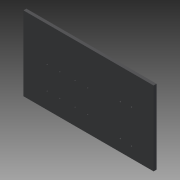
# Autodesk Inventor part: Base
Saved by Autodesk Inventor 2014 SP2 (Build 180246200, 246)
## iProperties
Created: 2015-09-24
Part Number: Base
Material: PVC, non plastifié
Document SubType Name: Modeling
Designer: sd
Density: 1.4 g/cm^3
Appearance: Gris
Mass: 783.12 g
Surface Area: 1491.46 cm^2
Volume: 559.372 cm^3
Author: sd
Autodesk Inventor part; units mm, degrees
ref_plane "YZ Plane" through (0, 0, 0) normal (1, 0, 0) x (0, 1, 0)
ref_plane "XZ Plane" through (0, 0, 0) normal (0, 1, 0) x (-1, 0, 0)
ref_plane "XY Plane" through (0, 0, 0) normal (0, 0, 1) x (1, 0, 0)
sketch "Esquisse1" plane through (0, 0, 0) normal (0, 1, 0) x (-1, 0, 0)
  line L0 (-180.6452, 101.6129) -> (169.3548, 101.6129)
  line L1 (169.3548, 101.6129) -> (169.3548, -98.3871)
  line L2 (169.3548, -98.3871) -> (-180.6452, -98.3871)
  line L3 (-180.6452, -98.3871) -> (-180.6452, 101.6129)
  point P0 (0, 0)
  dimension "d0" = 350
  dimension "d1" = 200
  constraints: 8 end point, 2 parallel, 1 horizontal, 1 perpendicular
  measures "d0" distance of L0.start L0.end
  measures "d1" distance of L2.end L0.start
extrude "Extrusion1" add sketch "Esquisse1" along normal blind 8
sketch "Esquisse2" plane through (0, 8, 0) normal (0, 1, 0) x (1, 0, 0)
  line L0 (180.6452, -101.6129) -> (180.6452, 98.3871) projected
  line L1 (180.6452, 98.3871) -> (-169.3548, 98.3871) projected
  circle A0 centre (120.6452, 68.3871) radius 2.5
  circle A1 centre (90.6452, 65.8871) radius 2.5
  circle A2 centre (120.6452, -22.6129) radius 2.5
  circle A3 centre (90.6452, -20.1129) radius 2.5
  point P0 (0, 0)
  dimension "d4" = 5
  dimension "d5" = 5
  dimension "d6" = 5
  dimension "d7" = 5
  dimension "d8" = 86
  dimension "d9" = 91
  dimension "d10" = 30
  dimension "d11" = 2.5
  dimension "d12" = 30
  dimension "d13" = 30
  dimension "d14" = 60
  dimension "d15" = 60
  constraints: 4 centre point
  measures "d4" diameter of A1
  measures "d5" diameter of A0
  measures "d6" diameter of A2
  measures "d7" diameter of A3
  measures "d8" distance of A3.centre A1.centre
  measures "d9" distance of A2.centre A0.centre
  measures "d10" horizontal distance of A1.centre A0.centre
  measures "d11" vertical distance of A2.centre A3.centre
  measures "d12" horizontal distance of A2.centre A3.centre
  measures "d13" distance from line of L1 A0.centre
  measures "d14" distance from line of L0 A0.centre
  measures "d15" distance from line of L0 A2.centre
extrude "Extrusion2" cut sketch "Esquisse2" against normal through all
sketch "Esquisse3" plane through (0, 8, 0) normal (0, 1, 0) x (1, 0, 0)
  circle A0 centre (90.6452, 65.8871) radius 2.5 projected
  circle A1 centre (90.6452, -20.1129) radius 2.5 projected
  line L0 (180.6452, 98.3871) -> (-169.3548, 98.3871) projected
  circle A2 centre (2.8852, 53.8871) radius 2
  circle A3 centre (-31.1148, 53.8871) radius 2
  circle A4 centre (-72.2148, 53.8871) radius 2
  circle A5 centre (-106.2148, 53.8871) radius 2
  circle A6 centre (-106.2148, -8.1129) radius 2
  circle A7 centre (-72.2148, -8.1129) radius 2
  circle A8 centre (-31.1148, -8.1129) radius 2
  circle A9 centre (2.8852, -8.1129) radius 2
  point P0 (0, 0)
  dimension "d18" = 4
  dimension "d19" = 4
  dimension "d20" = 4
  dimension "d21" = 4
  dimension "d22" = 4
  dimension "d23" = 4
  dimension "d24" = 4
  dimension "d25" = 4
  dimension "d26" = 62
  dimension "d27" = 62
  dimension "d28" = 62
  dimension "d29" = 62
  dimension "d30" = 34
  dimension "d31" = 34
  dimension "d32" = 34
  dimension "d33" = 34
  dimension "d34" = 41.1
  dimension "d35" = 41.1
  dimension "d36" = 87.76
  dimension "d37" = 87.76
  dimension "d38" = 32.5
  dimension "d39" = 86
  dimension "d40" = 44.5
  dimension "d41" = 44.5
  dimension "d42" = 44.5
  dimension "d43" = 44.5
  constraints: 8 centre point
  measures "d18" diameter of A5
  measures "d19" diameter of A4
  measures "d20" diameter of A3
  measures "d21" diameter of A2
  measures "d22" diameter of A9
  measures "d23" diameter of A8
  measures "d24" diameter of A7
  measures "d25" diameter of A6
  measures "d26" distance of A9.centre A2.centre
  measures "d27" distance of A8.centre A3.centre
  measures "d28" distance of A7.centre A4.centre
  measures "d29" distance of A6.centre A5.centre
  measures "d30" distance of A2.centre A3.centre
  measures "d31" distance of A9.centre A8.centre
  measures "d32" distance of A5.centre A4.centre
  measures "d33" distance of A7.centre A6.centre
  measures "d34" distance of A3.centre A4.centre
  measures "d35" distance of A8.centre A7.centre
  measures "d36" horizontal distance of A0.centre A2.centre
  measures "d37" horizontal distance of A1.centre A9.centre
  measures "d38" distance from line of L0 A0.centre
  measures "d39" distance of A1.centre A0.centre
  measures "d40" distance from line of A2.centre L0
  measures "d41" distance from line of L0 A3.centre
  measures "d42" distance from line of L0 A4.centre
  measures "d43" distance from line of L0 A5.centre
extrude "Extrusion3" cut sketch "Esquisse3" against normal through all contours A2 | A3 | A4 | A5 | A6 | A7 | A8 | A9
equation "\"d5\" = d4"
equation "\"d6\" = d4"
equation "\"d7\" = d4"
equation "\"d12\" = d10"
equation "\"d15\" = d14"
equation "\"d19\" = d18"
equation "\"d20\" = d18"
equation "\"d21\" = d18"
equation "\"d22\" = d18"
equation "\"d23\" = d18"
equation "\"d24\" = d18"
equation "\"d25\" = d18"
equation "\"d27\" = d26"
equation "\"d28\" = d26"
equation "\"d29\" = d26"
equation "\"d31\" = d30"
equation "\"d33\" = d32"
equation "\"d35\" = d34"
equation "\"d37\" = d36"
equation "\"d40\" = d38 + 0.5 * d39 - 0.5 * d26"
equation "\"d41\" = d40"
equation "\"d42\" = d40"
equation "\"d43\" = d40"
